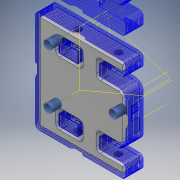
# Autodesk Inventor part: ptgrey_fix2
Saved by Autodesk Inventor 2018 (Build 220112000, 112)
## iProperties
Created: 2017-04-14
Part Number: ptgrey_fix2
Material: Aluminum 6061
Document SubType Name: Modeling
Designer: steve
Density: 2.7 g/cm^3
Appearance: Aluminum - Flat
Mass: 11.2958 g
Surface Area: 30.5005 cm^2
Volume: 4.18364 cm^3
Vendor: Rhoban
fix_width: 34,000 mm
side_fix_2_back: 4,650 mm
side_fix_spacing: 14,700 mm
side_fix_clearance: 5,000 mm
cam_fix_clearance: 8,000 mm
fix_length: 30,000 mm
thickness: 6,250 mm
Author: steve
Autodesk Inventor part; units mm, degrees
note: some values were not read from the file. Chosen so that the rebuilt part matches the saved one: direction of "Hole1".
ref_plane "YZ Plane" through (0, 0, 0) normal (1, 0, 0) x (0, 1, 0)
ref_plane "XZ Plane" through (0, 0, 0) normal (0, 1, 0) x (-1, 0, 0)
sketch "Sketch1" plane through (0, 0, 0) normal (0, 1, 0) x (-1, 0, 0)
  line L0 (-15, -17) -> (15, -17)
  line L1 (15, -17) -> (15, 17)
  line L2 (15, 17) -> (-15, 17)
  line L3 (-15, 17) -> (-15, -17)
  line L4 (-15, -17) -> (15, 17) construction
  line L5 (15, -17) -> (-15, 17) construction
  line L6 (-21, 0) -> (21, 0) construction
  line L7 (15, 10) -> (-15, 10) construction
  line L8 (11.85, 17) -> (11.85, -17) construction
  line L9 (0, -23.8) -> (0, 23.8) construction
  line L10 (-11.85, 17) -> (-11.85, -17) construction
  line L11 (15, -10) -> (-15, -10) construction
  circle A0 centre (11.85, 10) radius 1.5
  circle A1 centre (11.85, -10) radius 1.5
  circle A2 centre (-11.85, 0) radius 1.5
  point P0 (0, 0)
  dimension "d0" = 34
  dimension "d1" = 30
  dimension "d2" = 10
  dimension "d3" = 11.85
  dimension "d4" = 3
  dimension "d5" = 3
  dimension "d6" = 3
  constraints: 20 end point, 9 point on line, 4 symmetric about line, 3 centre point, 3 midpoint, 2 horizontal, 2 parallel, 1 perpendicular, 1 vertical
  measures "d0" distance of L0.end L1.end
  measures "d1" distance of L0.start L0.end
  measures "d2" distance between parallel lines of L6 L7
  measures "d3" distance between parallel lines of L8 L9
  measures "d4" diameter of A0
  measures "d5" diameter of A1
  measures "d6" diameter of A2
extrude "Extrusion1" add sketch "Sketch1" along normal blind 3.25
sketch "Sketch2" plane through (0, 3.25, 0) normal (0, 1, 0) x (1, 0, 0)
  line L0 (15, 17) -> (-15, 17) projected
  line L1 (15, -17) -> (15, 17) projected
  line L2 (-15, 17) -> (15, 17)
  line L3 (15, 17) -> (15, 15)
  line L4 (15, 15) -> (-15, 15)
  line L5 (-15, 15) -> (-15, 17)
  line L6 (21, 0) -> (-21, 0) construction
  line L7 (15, -17) -> (-15, -17)
  line L8 (15, 17) -> (15, -17)
  line L9 (15, -15) -> (-15, -15)
  line L10 (-15, -15) -> (-15, -17)
  point P0 (0, 0)
  dimension "d9" = 2
  constraints: 16 end point, 5 symmetric about line, 2 parallel, 2 point on line, 1 horizontal, 1 perpendicular
  measures "d9" distance between parallel lines of L0 L4
extrude "Extrusion2" add sketch "Sketch2" along normal blind 3
sketch "Sketch5" plane through (15, 0, -17) normal (0, 0, -1) x (-1, 0, 0)
  line L0 (0, 0) -> (30, 0) projected
  line L1 (30, 0) -> (30, 6.25) projected
  line L2 (0, 6.25) -> (30, 6.25) projected
  line L3 (0, 0) -> (0, 6.25) projected
  line L4 (0, 3.125) -> (4.65, 3.125) construction
  line L5 (4.65, 3.125) -> (19.35, 3.125) construction
  dimension "d40" = 4.65
  dimension "d41" = 14.7
  constraints: 4 end point, 2 coincident, 2 horizontal, 1 midpoint
  measures "d40" distance of L4.start L4.end
  measures "d41" distance of L4.end L5.end
sketch "Sketch8" plane through (0, 3.25, 0) normal (0, 1, 0) x (1, 0, 0)
  line L0 (15, 15) -> (-15, 15) projected
  line L1 (-15, 15) -> (-15, -15) projected
  line L2 (-15, -15) -> (15, -15) projected
  line L3 (15, -15) -> (15, 15) projected
  circle A0 centre (-11.85, -10) radius 1.5 projected
  circle A1 centre (-11.85, 10) radius 1.5 projected
  circle A2 centre (11.85, 0) radius 1.5 projected
  line L4 (-9.35, -15) -> (-9.35, -8)
  line L5 (-9.35, -8) -> (0.65, -8)
  line L6 (0.65, -8) -> (0.65, -15)
  line L7 (15, -8) -> (5.35, -8)
  line L8 (5.35, -8) -> (5.35, -15)
  line L9 (15, -8) -> (15, -15)
  line L10 (15, -17) -> (15, 17) projected
  line L11 (15, -15) -> (5.35, -15)
  line L12 (0.65, -15) -> (-9.35, -15)
  line L13 (15, 0) -> (-15, 0) construction
  line L14 (-15, 17) -> (-15, -17) construction
  line L15 (-15, 15) -> (15, 15)
  line L16 (15, 15) -> (15, -15)
  line L17 (-9.35, 15) -> (-9.35, 8)
  line L18 (-9.35, 8) -> (0.65, 8)
  line L19 (0.65, 8) -> (0.65, 15)
  line L20 (15, 8) -> (5.35, 8)
  line L21 (5.35, 8) -> (5.35, 15)
  line L22 (15, 8) -> (15, 15)
  line L23 (15, 17) -> (15, -17)
  line L24 (15, 15) -> (5.35, 15)
  line L25 (0.65, 15) -> (-9.35, 15)
  circle A3 centre (11.85, 0) radius 4
  circle A4 centre (-11.85, 10) radius 4
  circle A5 centre (-11.85, -10) radius 4
  point P0 (0, 0)
  dimension "d34" = 9.65
  dimension "d35" = 4.7
  dimension "d36" = 10
  dimension "d37" = 8
  dimension "d44" = 8
  constraints: 40 end point, 12 point on line, 11 symmetric about line, 3 centre point, 3 coincident, 3 collinear, 3 perpendicular, 2 equal radius, 2 midpoint, 1 vertical
  measures "d34" distance between parallel lines of L3 L8
  measures "d35" distance between parallel lines of L6 L8
  measures "d36" distance between parallel lines of L4 L6
  measures "d37" distance from line of L7 A2.centre
  measures "d44" diameter of A3
extrude "Extrusion5" cut sketch "Sketch8" against normal through all contours L3 L20 L21 L0 | L19 L18 A4 L17 L0 | A4 L18 L17 | L3 L2 L8 L7 | A5 L4 L5 | L5 L6 L2 L4 A5
hole "Hole1" at (-4.35, 3.125, -17) at (10.35, 3.125, -17) direction (0, 0, 1) diameter 2.5 end up to surface
ref_plane "Work Plane1" through (15, 0, 0) normal (0, 0, -1) x (-1, 0, 0)
mirror "Mirror1" about plane through (15, 0, 0) normal (0, 0, -1) of "Hole1"
extrude "Extrusion6" add sketch "Sketch8" along normal blind 3 contours L21 L20 L3 A3 L7 L8 L2 L6 L5 A5 L1 A4 L18 L19 L0 | L3 A3 | L17 A4 L1 L0 | L17 L18 A4 L1 | A5 L5 L4 L1 | A5 L4 L2 L1 picked at (14.45, 0)
extrude "Extrusion7" cut sketch "Sketch8" along normal through all contours A3 L3 | L3 A3 | A4 L18 L17 | L17 L18 A4 L1 | L1 A4 | A5 L5 L4 L1 | L1 A5 | A5 L4 L5
fillet "Fillet3" radius 1.5 12 edges at (-9.35, 3.125, 15) (0.65, 3.125, -8) (-9.35, 1.625, -8) (5.35, 3.125, -8) (5.35, 3.125, 8) (-9.35, 1.625, 8) (0.65, 3.125, 8) (-9.35, 3.125, -15) (0.65, 3.125, -15) (5.35, 3.125, -15) (5.35, 3.125, 15) (0.65, 3.125, 15)
fillet "Fillet4" radius 1.5 2 edges at (15, 3.125, 8) (15, 3.125, -8)
equation "\"d0\" = fix_width"
equation "\"d1\" = fix_length"
equation "\"d7\" = first_layer_thickness"
equation "\"d10\" = thickness - first_layer_thickness"
equation "\"d40\" = side_fix_2_back"
equation "\"d41\" = side_fix_spacing"
equation "\"d34\" = side_fix_2_back + side_fix_clearance"
equation "\"d35\" = side_fix_spacing - 2 * side_fix_clearance"
equation "\"d36\" = 2 * side_fix_clearance"
equation "\"d37\" = cam_fix_clearance"
equation "\"d45\" = thickness - first_layer_thickness"
equation "\"d47\" = thickness - first_layer_thickness"
equation "\"fix_width\" = 34"
equation "\"side_fix_2_back\" = 4.65"
equation "\"side_fix_spacing\" = 14.7"
equation "\"side_fix_clearance\" = 5"
equation "\"cam_fix_clearance\" = 8"
equation "\"fix_length\" = 30"
equation "\"thickness\" = 6.25"
equation "\"first_layer_thickness\" = 3.25"
body "Solid1"
